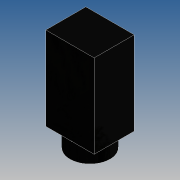
# Autodesk Inventor part: R006
Saved by Autodesk Inventor 2017 (Build 210142000, 142)
## iProperties
Created: 2018-11-02
Part Number: R006
Material: Générique
Document SubType Name: Modeling
Designer: Gilles Mottiez
Density: 1 g/cm^3
Appearance: Anodisé - Noir
Description: Port Jack Raspberry pi 3B
Author: Gilles Mottiez
Autodesk Inventor part; units mm, degrees
ref_plane "YZ Plane" through (0, 0, 0) normal (1, 0, 0) x (0, 1, 0)
ref_plane "XZ Plane" through (0, 0, 0) normal (0, 1, 0) x (-1, 0, 0)
ref_plane "XY Plane" through (0, 0, 0) normal (0, 0, 1) x (1, 0, 0)
sketch "Sketch1" plane through (0, 0, 0) normal (0, 0, 1) x (1, 0, 0)
  circle A0 centre (0, 0) radius 3
  circle A1 centre (0, 0) radius 2
  dimension "d0" = 6
  dimension "d1" = 4
  constraints: 2 centre point, 2 coincident
  measures "d0" diameter of A0
  measures "d1" diameter of A1
extrude "Extrusion1" add sketch "Sketch1" along normal blind 2.45
sketch "Esquisse2" plane through (0, 0, 2.45) normal (0, 0, 1) x (1, 0, 0)
  line L0 (-3.625, 3) -> (3.625, 3)
  line L1 (3.625, 3) -> (3.625, -3)
  line L2 (3.625, -3) -> (-3.625, -3)
  line L3 (-3.625, -3) -> (-3.625, 3)
  circle A0 centre (0, 0) radius 2 construction
  circle A1 centre (0, 0) radius 3 construction
  line L4 (0, 0) -> (0, 3) construction
  line L5 (0, 0) -> (0, -3) construction
  dimension "d4" = 7.25
  constraints: 12 end point, 2 horizontal alignment, 2 parallel, 2 point on circle, 2 vertical, 1 horizontal, 1 perpendicular, 1 other
  measures "d4" distance of L1.end L2.end
extrude "Extrusion2" add sketch "Esquisse2" along normal blind 12.5
